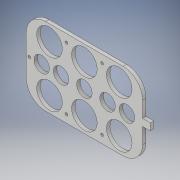
# Autodesk Inventor part: Bandeja de tubos
Saved by Autodesk Inventor 2017 (Build 210142000, 142)
## iProperties
Created: 2016-07-16
Part Number: Bandeja de tubos
Material: Generic
Document SubType Name: Modeling
Designer: mateu
Density: 1 g/cm^3
Appearance: Default
Author: mateu
Autodesk Inventor part; units mm, degrees
ref_plane "YZ Plane" through (0, 0, 0) normal (1, 0, 0) x (0, 1, 0)
ref_plane "XZ Plane" through (0, 0, 0) normal (0, 1, 0) x (-1, 0, 0)
ref_plane "XY Plane" through (0, 0, 0) normal (0, 0, 1) x (1, 0, 0)
sketch "Sketch1" plane through (0, 0, 0) normal (0, 0, 1) x (1, 0, 0)
  line L0 (0, 0) -> (150, 0)
  line L1 (150, 0) -> (150, -100)
  line L2 (150, -100) -> (0, -100)
  line L3 (0, -100) -> (0, 0)
  circle A0 centre (30, -20) radius 16.5
  circle A1 centre (30, -80) radius 16.5
  circle A2 centre (75, -20) radius 16.5
  circle A3 centre (120, -20) radius 16.5
  circle A4 centre (75, -80) radius 16.5
  circle A5 centre (120, -80) radius 16.5
  circle A6 centre (20, -50) radius 10
  circle A7 centre (45, -50) radius 10
  circle A8 centre (75, -50) radius 10
  circle A9 centre (105, -50) radius 10
  circle A10 centre (130, -50) radius 10
  circle A11 centre (52, -10) radius 1.75
  circle A12 centre (98, -10) radius 1.75
  circle A13 centre (52, -90) radius 1.75
  circle A14 centre (98, -90) radius 1.75
  circle A15 centre (4, -50) radius 1.75
  dimension "d0" = 150
  dimension "d1" = 100
  dimension "d2" = 33
  dimension "d3" = 33
  dimension "d5" = 33
  dimension "d6" = 33
  dimension "d8" = 33
  dimension "d9" = 33
  dimension "d10" = 20
  dimension "d11" = 20
  dimension "d12" = 20
  dimension "d13" = 30
  dimension "d14" = 30
  dimension "d15" = 75
  dimension "d16" = 30
  dimension "d17" = 75
  dimension "d18" = 30
  dimension "d19" = 20
  dimension "d20" = 20
  dimension "d21" = 20
  dimension "d22" = 20
  dimension "d23" = 20
  dimension "d25" = 20
  dimension "d26" = 20
  dimension "d27" = 20
  dimension "d28" = 20
  dimension "d29" = 20
  dimension "d30" = 25
  dimension "d31" = 25
  dimension "d32" = 50
  dimension "d33" = 50
  dimension "d34" = 50
  dimension "d35" = 50
  dimension "d36" = 50
  dimension "d37" = 75
  dimension "d56" = 3.5
  dimension "d57" = 3.5
  dimension "d58" = 3.5
  dimension "d59" = 3.5
  dimension "d60" = 10
  dimension "d61" = 10
  dimension "d62" = 10
  dimension "d63" = 10
  dimension "d64" = 52
  dimension "d65" = 52
  dimension "d66" = 52
  dimension "d67" = 52
  dimension "d74" = 3.5
  dimension "d75" = 4
  dimension "d76" = 50
  constraints: 16 centre point, 8 end point, 2 parallel, 1 horizontal, 1 perpendicular
  measures "d0" distance of L1.end L2.end
  measures "d1" distance of L0.end L1.end
  measures "d2" diameter of A0
  measures "d3" diameter of A1
  measures "d5" diameter of A2
  measures "d6" diameter of A3
  measures "d8" diameter of A4
  measures "d9" diameter of A5
  measures "d10" distance from line of L2 A1.centre
  measures "d11" distance from line of L2 A4.centre
  measures "d12" distance from line of L2 A5.centre
  measures "d13" distance from line of L3 A1.centre
  measures "d14" distance from line of L1 A5.centre
  measures "d15" distance from line of L1 A4.centre
  measures "d16" distance from line of L3 A0.centre
  measures "d17" distance from line of L3 A2.centre
  measures "d18" distance from line of L1 A3.centre
  measures "d19" distance from line of L0 A0.centre
  measures "d20" distance from line of L0 A2.centre
  measures "d21" distance from line of L0 A3.centre
  measures "d22" diameter of A6
  measures "d23" diameter of A7
  measures "d25" diameter of A8
  measures "d26" diameter of A9
  measures "d27" diameter of A10
  measures "d28" distance from line of L3 A6.centre
  measures "d29" distance from line of L1 A10.centre
  measures "d30" distance of A6.centre A7.centre
  measures "d31" distance of A10.centre A9.centre
  measures "d32" distance from line of L2 A8.centre
  measures "d33" distance from line of L2 A9.centre
  measures "d34" distance from line of L2 A10.centre
  measures "d35" distance from line of L2 A7.centre
  measures "d36" distance from line of L2 A6.centre
  measures "d37" distance from line of L3 A8.centre
  measures "d56" diameter of A11
  measures "d57" diameter of A12
  measures "d58" diameter of A13
  measures "d59" diameter of A14
  measures "d60" distance from line of L2 A14.centre
  measures "d61" distance from line of L2 A13.centre
  measures "d62" distance from line of L0 A11.centre
  measures "d63" distance from line of L0 A12.centre
  measures "d64" distance from line of L3 A11.centre
  measures "d65" distance from line of L1 A12.centre
  measures "d66" distance from line of L1 A14.centre
  measures "d67" distance from line of L3 A13.centre
  measures "d74" diameter of A15
  measures "d75" distance from line of L3 A15.centre
  measures "d76" distance from line of L2 A15.centre
extrude "Extrusion5" add sketch "Sketch1" along normal blind 4.5
sketch "Sketch4" plane through (150, -100, 0) normal (1, 0, 0) x (0, 0, -1)
  line L0 (0, 0) -> (-4.5, 0) projected
  line L1 (0, 100) -> (-4.5, 100)
  line L2 (-4.5, 100) -> (-4.5, 0)
  line L3 (-4.5, 0) -> (0, 0)
  line L4 (0, 0) -> (0, 100)
  line L5 (-4.5, 40) -> (-4.5, 60) projected
  line L6 (-4.5, 45.5) -> (0, 45.5)
  line L7 (0, 45.5) -> (0, 54.5)
  line L8 (0, 54.5) -> (-4.5, 54.5)
  line L9 (-4.5, 54.5) -> (-4.5, 45.5)
  dimension "d79" = 9
  dimension "d80" = 45.5
  constraints: 16 end point, 4 parallel, 2 horizontal, 2 perpendicular, 2 point on line
  measures "d79" distance of L7.end L6.end
  measures "d80" distance between parallel lines of L1 L8
extrude "Extrusion6" add sketch "Sketch4" along normal blind 10 contours L6 L2 L8 L4
fillet "Fillet9" radius 25 1 edges at (150, 0, 2.25)
fillet "Fillet10" radius 25 1 edges at (150, -100, 2.25)
fillet "Fillet11" radius 25 1 edges at (0, -100, 2.25)
fillet "Fillet12" radius 25 1 edges at (0, 0, 2.25)
body "Solid3"
